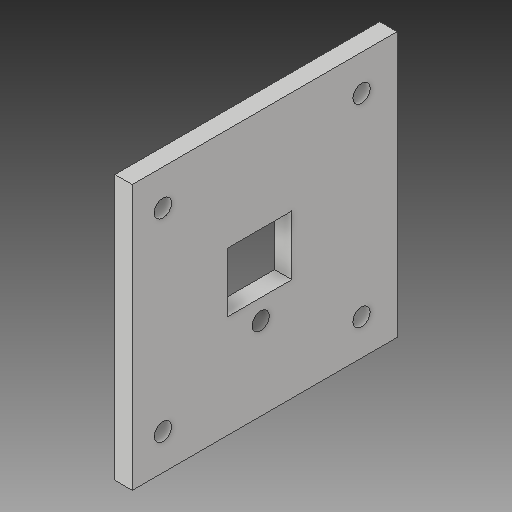
# Autodesk Inventor part: plateform du bas
Saved by Autodesk Inventor 2017 (Build 210142000, 142)
## iProperties
Created: 2018-11-16
Part Number: plateform du bas
Material: Generic
Document SubType Name: Modeling
Designer: Antoine Blaud
Density: 1 g/cm^3
Appearance: Default
Author: Antoine Blaud
Autodesk Inventor part; units mm, degrees
ref_plane "YZ Plane" through (0, 0, 0) normal (1, 0, 0) x (0, 1, 0)
ref_plane "XZ Plane" through (0, 0, 0) normal (0, 1, 0) x (-1, 0, 0)
ref_plane "XY Plane" through (0, 0, 0) normal (0, 0, 1) x (1, 0, 0)
sketch "Sketch1" plane through (0, 0, 0) normal (1, 0, 0) x (0, 1, 0)
  line L0 (0, 0) -> (76.2, 0)
  line L1 (76.2, 0) -> (76.2, -76.2)
  line L2 (76.2, -76.2) -> (0, -76.2)
  line L3 (0, -76.2) -> (0, 0)
  line L4 (20.4851, -17.6149) -> (55.7149, -17.6149)
  line L5 (55.7149, -17.6149) -> (55.7149, -55.7149)
  line L6 (55.7149, -55.7149) -> (20.4851, -55.7149)
  line L7 (20.4851, -55.7149) -> (20.4851, -17.6149)
  line L8 (20.4851, -17.6149) -> (55.7149, -55.7149) construction
  line L9 (55.7149, -17.6149) -> (20.4851, -55.7149) construction
  line L10 (76.2, 0) -> (55.7149, -17.6149)
  line L11 (20.4851, -55.7149) -> (0, -76.2)
  line L12 (0, 0) -> (20.4851, -17.6149)
  line L13 (55.7149, -55.7149) -> (76.2, -76.2)
  circle A0 centre (65.9575, -8.8074) radius 2.5
  circle A1 centre (65.9575, -65.9574) radius 2.5
  circle A2 centre (10.2426, -65.9575) radius 2.5
  circle A3 centre (10.2426, -8.8074) radius 2.5
  line L14 (29.5453, -27.4133) -> (46.6547, -27.4133)
  line L15 (46.6547, -27.4133) -> (46.6547, -45.9165)
  line L16 (46.6547, -45.9165) -> (29.5453, -45.9165)
  line L17 (29.5453, -45.9165) -> (29.5453, -27.4133)
  line L18 (29.5453, -27.4133) -> (46.6547, -45.9165) construction
  line L19 (46.6547, -27.4133) -> (29.5453, -45.9165) construction
  point P0 (38.1, -36.6649)
  dimension "d0" = 76.2
  dimension "d1" = 76.2
  dimension "d2" = 35.2298
  dimension "d3" = 38.1
  dimension "d4" = 5
  dimension "d5" = 5
  dimension "d6" = 5
  dimension "d7" = 5
  dimension "d8" = 49.308
  dimension "d9" = 29.5453
  constraints: 40 end point, 8 midpoint, 6 parallel, 4 centre point, 4 perpendicular, 3 horizontal, 1 point on line
  measures "d0" distance between parallel lines of L1 L3
  measures "d1" distance between parallel lines of L0 L2
  measures "d2" distance of L5.end L6.end
  measures "d3" distance of L4.end L5.end
  measures "d4" diameter of A0
  measures "d5" diameter of A1
  measures "d6" diameter of A2
  measures "d7" diameter of A3
  measures "d8" angle of L10 L1
  measures "d9" distance between parallel lines of L15 L1
extrude "Extrusion1" add sketch "Sketch1" along normal blind 5
extrude "Extrusion2" cut sketch "Sketch1" along normal blind 5 contours A3 L12 | L12 A3 | A0 L10 | L10 A0 | A2 L11 | L11 A2 | A1 L13 | L13 A1
sketch "Sketch2" plane through (5, 0, 0) normal (1, 0, 0) x (0, 0, -1)
  line L0 (76.2, 0) -> (76.2, 76.2) projected
  line L1 (27.4133, 29.5453) -> (76.2, 0)
  line L2 (45.9165, 29.5453) -> (0, 0)
  circle A0 centre (36.9453, 23.7727) radius 2.5
  line L3 (36.9453, 23.7727) -> (36.9453, 0)
  dimension "d14" = 5
  dimension "d19" = 23.7727
  constraints: 6 end point, 2 point on line, 1 centre point, 1 vertical
  measures "d14" diameter of A0
  measures "d19" distance of L3.start L3.end
extrude "Extrusion3" cut sketch "Sketch2" against normal blind 25.4
thread "Thread1" size "M1x0.25" class "6H" standard "ISO Metric profile" full length
body "Solid1"
